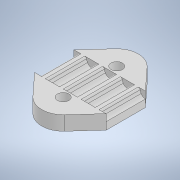
# Autodesk Inventor part: ベルト固定_3Dプリンタ
Saved by Autodesk Inventor 2021 (Build 250183000, 183)
## iProperties
Created: 2022-02-24
Part Number: ベルト固定_3Dプリンタ
Material: 一般
Document SubType Name: Modeling
Designer: hirohumi
Density: 1 g/cm^3
Appearance: 既定
Author: hirohumi
Autodesk Inventor part; units mm, degrees
ref_plane "YZ Plane" through (0, 0, 0) normal (1, 0, 0) x (0, 1, 0)
ref_plane "XZ Plane" through (0, 0, 0) normal (0, 1, 0) x (-1, 0, 0)
ref_plane "XY Plane" through (0, 0, 0) normal (0, 0, 1) x (1, 0, 0)
sketch "スケッチ1" plane through (0, 0, 0) normal (0, 0, 1) x (1, 0, 0)
  arc A0 (-1.2061, 2.7902) -> (0, 2.07) centre (0, 3.44) ccw construction
  arc A1 (-1.4749, 3.5744) -> (-1.2061, 2.7902) centre (1.03, 3.995) ccw construction
  arc A2 (1.2061, 2.7902) -> (1.4749, 3.5744) centre (-1.03, 3.995) ccw
  arc A3 (-1.4749, 3.5744) -> (-1.9779, 4) centre (-1.9779, 3.49) ccw construction
  arc A4 (1.9779, 4) -> (1.4749, 3.5744) centre (1.9779, 3.49) ccw
  line L0 (1.9779, 4) -> (2.5, 4)
  line L1 (-1.9779, 4) -> (-2.5, 4) construction
  line L2 (6.9779, 4) -> (7.5, 4)
  arc A5 (6.9779, 4) -> (6.4749, 3.5744) centre (6.9779, 3.49) ccw
  arc A6 (6.2061, 2.7902) -> (6.4749, 3.5744) centre (3.97, 3.995) ccw
  arc A7 (3.7939, 2.7902) -> (6.2061, 2.7902) centre (5, 3.44) ccw
  arc A8 (3.5251, 3.5744) -> (3.7939, 2.7902) centre (6.03, 3.995) ccw
  arc A9 (3.5251, 3.5744) -> (3.0221, 4) centre (3.0221, 3.49) ccw
  line L3 (3.0221, 4) -> (2.5, 4)
  line L4 (11.9779, 4) -> (12.5, 4)
  arc A10 (11.9779, 4) -> (11.4749, 3.5744) centre (11.9779, 3.49) ccw
  arc A11 (11.2061, 2.7902) -> (11.4749, 3.5744) centre (8.97, 3.995) ccw
  arc A12 (8.7939, 2.7902) -> (11.2061, 2.7902) centre (10, 3.44) ccw
  arc A13 (8.5251, 3.5744) -> (8.7939, 2.7902) centre (11.03, 3.995) ccw
  arc A14 (8.5251, 3.5744) -> (8.0221, 4) centre (8.0221, 3.49) ccw
  line L5 (8.0221, 4) -> (7.5, 4)
  line L6 (16.9779, 4) -> (17.5, 4)
  arc A15 (16.9779, 4) -> (16.4749, 3.5744) centre (16.9779, 3.49) ccw
  arc A16 (16.2061, 2.7902) -> (16.4749, 3.5744) centre (13.97, 3.995) ccw
  arc A17 (13.7939, 2.7902) -> (16.2061, 2.7902) centre (15, 3.44) ccw
  arc A18 (13.5251, 3.5744) -> (13.7939, 2.7902) centre (16.03, 3.995) ccw
  arc A19 (13.5251, 3.5744) -> (13.0221, 4) centre (13.0221, 3.49) ccw
  line L7 (13.0221, 4) -> (12.5, 4)
  line L8 (21.9779, 4) -> (22.5, 4) construction
  arc A20 (21.9779, 4) -> (21.4749, 3.5744) centre (21.9779, 3.49) ccw construction
  arc A21 (21.2061, 2.7902) -> (21.4749, 3.5744) centre (18.97, 3.995) ccw construction
  arc A22 (18.7939, 2.7902) -> (20, 2.07) centre (20, 3.44) ccw
  arc A23 (18.5251, 3.5744) -> (18.7939, 2.7902) centre (21.03, 3.995) ccw
  arc A24 (18.5251, 3.5744) -> (18.0221, 4) centre (18.0221, 3.49) ccw
  line L9 (18.0221, 4) -> (17.5, 4)
  line L10 (0, 2.07) -> (0, 0)
  line L11 (0, 0) -> (20, 0)
  line L12 (20, 0) -> (20, 2.07)
  arc A25 (0, 2.07) -> (1.2061, 2.7902) centre (0, 3.44) ccw
  arc A26 (20, 2.07) -> (21.2061, 2.7902) centre (20, 3.44) ccw construction
  point P0 (5, 2.07)
  point P1 (10, 2.07)
  point P2 (15, 2.07)
  point P3 (22.5, 4)
  dimension "d9" = 1.37
  dimension "d10" = 2.54
  dimension "d11" = 2.54
  dimension "d12" = 0.51
  dimension "d13" = 0.51
  dimension "d14" = 1.93
  dimension "d15" = 5
  dimension "d16" = 2.5
  dimension "d17" = 5
  constraints: 54 point on circle, 27 centre point, 26 end point, 6 tangent, 2 horizontal, 2 perpendicular, 1 horizontal alignment, 1 vertical, 1 vertical alignment
  measures "d9" radius of A0
  measures "d10" radius of A1
  measures "d11" radius of A2
  measures "d12" radius of A3
  measures "d13" radius of A4
  measures "d14" distance from line of L0 L10.start
  measures "d15" distance of L0.end L1.end
  measures "d16" horizontal distance of A0.centre L1.end
  measures "d17" distance of L0.end L2.end
extrude "押し出し1" add sketch "スケッチ1" along normal blind 11
sketch "スケッチ5" plane through (0, 0, 0) normal (0, -1, 0) x (1, 0, 0)
  circle A0 centre (10, 13) radius 1.6
  circle A1 centre (10, -2) radius 1.6
  arc A2 (14.413, 17.0651) -> (5.587, 17.0651) centre (10, 13) ccw
  arc A3 (5.587, -6.0651) -> (14.413, -6.0651) centre (10, -2) ccw
  line L0 (0, 11) -> (20, 11) projected
  line L1 (20, 11) -> (14.413, 17.0651)
  line L2 (5.587, 17.0651) -> (0, 11)
  line L3 (0, 0) -> (20, 0) projected
  line L4 (20, 0) -> (14.413, -6.0651)
  line L5 (5.587, -6.0651) -> (0, 0)
  point P0 (10, 11)
  point P1 (10, 0)
  dimension "d30" = 3.2
  dimension "d31" = 3.2
  dimension "d32" = 6
  dimension "d33" = 6
  dimension "d34" = 2
  dimension "d35" = 2
  constraints: 8 end point, 4 centre point, 4 point on circle, 4 tangent, 2 coincident, 2 midpoint, 2 vertical alignment
  measures "d30" diameter of A0
  measures "d31" diameter of A1
  measures "d32" radius of A2
  measures "d33" radius of A3
  measures "d34" distance from line of L3 A1.centre
  measures "d35" distance from line of L0 A0.centre
extrude "押し出し5" add sketch "スケッチ5" against normal blind 4
